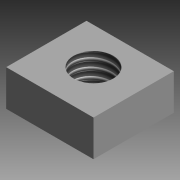
# Autodesk Inventor part: mutter
Saved by Autodesk Inventor 2013 (Build 170138000, 138)
## iProperties
Created: 2012-10-24
Part Number: mutter
Material: Allgemein
Document SubType Name: Modeling
Designer: fivef
Density: 1 g/cm^3
Author: fivef
Autodesk Inventor part; units mm, degrees
ref_plane "YZ Plane" through (0, 0, 0) normal (1, 0, 0) x (0, 1, 0)
ref_plane "XZ Plane" through (0, 0, 0) normal (0, 1, 0) x (-1, 0, 0)
ref_plane "XY Plane" through (0, 0, 0) normal (0, 0, 1) x (1, 0, 0)
sketch "Skizze1" plane through (0, 0, 0) normal (0, 0, 1) x (1, 0, 0)
  line L0 (3.75, 4.9488) -> (3.75, -1.9512) projected
  line L1 (-3.75, -1.9512) -> (-3.75, 4.9488) projected
  line L2 (3.75, -1.9512) -> (-3.75, -1.9512) projected
  line L3 (0, 0) -> (3.75, 0) construction
  line L4 (0, 1.7988) -> (0, -1.9512) construction
  line L5 (-3.75, 4.9488) -> (3.75, 4.9488)
  line L6 (3.75, 4.9488) -> (3.75, -1.9512)
  line L7 (3.75, -1.9512) -> (-3.75, -1.9512)
  line L8 (-3.75, -1.9512) -> (-3.75, 4.9488)
  circle A0 centre (0, 1.7988) radius 1.7
  dimension "d0" = 3.75
  dimension "d2" = 3.75
  dimension "d5" = 3.4
  constraints: 12 end point, 3 parallel, 1 centre point, 1 horizontal, 1 midpoint, 1 perpendicular
  measures "d0" distance of L3.start L3.end
  measures "d2" distance of L4.start L4.end
  measures "d5" diameter of A0
extrude "Extrusion2" add sketch "Skizze1" against normal blind 3.1
thread "Gewinde1" size "M4x0.7" class "6H" standard "ANSI Metric M Profile" full length
